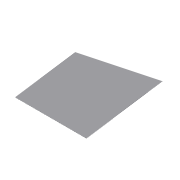
# Autodesk Inventor part: panelCflat.KR
Saved by Autodesk Inventor 2016 (Build 200138000, 138)
## iProperties
Created: 2015-02-12
Part Number: panelCflat.KR
Material: Generic
Document SubType Name: Modeling
Designer: Dave
Density: 1 g/cm^3
Appearance: Default
Author: Dave
Autodesk Inventor part; units mm, degrees
ref_plane "YZ Plane" through (0, 0, 0) normal (1, 0, 0) x (0, 1, 0)
ref_plane "XZ Plane" through (0, 0, 0) normal (0, 1, 0) x (-1, 0, 0)
ref_plane "XY Plane" through (0, 0, 0) normal (0, 0, 1) x (1, 0, 0)
sketch "Sketch1" plane through (0, 0, 0) normal (0, 1, 0) x (-1, 0, 0)
  line L0 (0, 0) -> (-12922.0343, 0) construction
  line L1 (0, 0) -> (-12360.1465, -3311.8913) construction
  line L2 (0, 0) -> (13412.8311, 0) construction
  line L3 (-4192.3928, 50) -> (-5412.3928, 50)
  line L4 (-4036.5995, -1133.3674) -> (-5215.029, -1449.1266)
  line L5 (-4036.5995, -1133.3674) -> (-4192.3928, 50)
  line L6 (0, 0) -> (-4114.4962, -541.6837) construction
  line L7 (0, 0) -> (4150, 0) construction
  line L8 (-5412.3928, 50) -> (-5215.029, -1449.1266)
  dimension "d0" = 165
  dimension "d3" = 50
  dimension "d4" = 50
  dimension "d6" = 4150
  dimension "d7" = 172.5
  dimension "d10" = 1220
  constraints: 20 end point, 3 horizontal, 3 parallel, 1 equal length, 1 midpoint, 1 perpendicular
  measures "d0" angle of L1 L2
  measures "d3" distance between parallel lines of L3 L0
  measures "d4" distance between parallel lines of L1 L4
  measures "d6" distance of L6.end L0.start
  measures "d7" angle of L6 L7
  measures "d10" distance of L3.end L3.start
extrude "Extrusion1" add sketch "Sketch1" along normal blind 1
body "Solid1"
